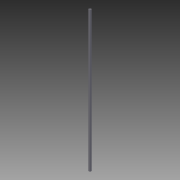
# Autodesk Inventor part: Robot-Mast
Saved by Autodesk Inventor 2012 (Build 160160000, 160)
## iProperties
Created: 2013-07-14
Part Number: Robot-Mast
Material: Aluminum-6061
Document SubType Name: Modeling
Designer: joe_000
Density: 2.71 g/cm^3
Mass: 507.328 g
Surface Area: 2108.26 cm^2
Volume: 187.206 cm^3
MastWidth: 0.750 in
Author: joe_000
Autodesk Inventor part; units mm, degrees
ref_plane "YZ Plane" through (0, 0, 0) normal (1, 0, 0) x (0, 1, 0)
ref_plane "XZ Plane" through (0, 0, 0) normal (0, 1, 0) x (-1, 0, 0)
ref_plane "XY Plane" through (0, 0, 0) normal (0, 0, 1) x (1, 0, 0)
sketch "Sketch1" plane through (0, 0, 0) normal (0, 1, 0) x (-1, 0, 0)
  line L0 (0, 0) -> (19.05, 0)
  line L1 (19.05, 0) -> (19.05, 19.05)
  line L2 (19.05, 19.05) -> (0, 19.05)
  line L3 (0, 19.05) -> (0, 0)
  line L4 (1.778, 17.272) -> (17.272, 17.272)
  line L5 (17.272, 17.272) -> (17.272, 1.778)
  line L6 (17.272, 1.778) -> (1.778, 1.778)
  line L7 (1.778, 1.778) -> (1.778, 17.272)
  dimension "MastWidth" = 19.05
  dimension "d1" = 19.05
  dimension "d2" = 1.778
  dimension "d3" = 1.778
  dimension "d4" = 1.778
  dimension "d5" = 1.778
  constraints: 16 end point, 4 parallel, 2 horizontal, 2 perpendicular
  measures "MastWidth" distance of L1.end L2.end
  measures "d1" distance of L0.end L1.end
  measures "d2" distance between parallel lines of L2 L4
  measures "d3" distance between parallel lines of L3 L7
  measures "d4" distance between parallel lines of L0 L6
  measures "d5" distance between parallel lines of L1 L5
extrude "Extrusion1" add sketch "Sketch1" along normal blind 1524
sketch "Sketch2" plane through (0, 0, 0) normal (0, -1, 0) x (1, 0, 0)
  line L0 (-17.272, 1.778) -> (-17.272, 17.272) projected
  line L1 (-17.272, 17.272) -> (-1.778, 17.272) projected
  line L2 (-1.778, 17.272) -> (-1.778, 1.778) projected
  line L3 (-1.778, 1.778) -> (-17.272, 1.778) projected
  line L4 (0, 0) -> (-19.05, 0) projected
  line L5 (0, 19.05) -> (0, 0) projected
  line L6 (-19.05, 19.05) -> (0, 19.05) projected
  line L7 (-19.05, 0) -> (-19.05, 19.05) projected
  line L8 (-19.05, 9.525) -> (0, 9.525)
  line L9 (-9.525, 19.05) -> (-9.525, 0)
  constraints: 4 end point, 4 midpoint
sketch "Sketch3" plane through (-19.05, 0, 19.05) normal (0, 0, 1) x (1, 0, 0)
  line L0 (19.05, 1524) -> (0, 1524) projected
  line L1 (0, 0) -> (0, 1524) projected
  line L2 (0, 0) -> (19.05, 0) projected
  line L3 (19.05, 0) -> (19.05, 1524) projected
  line L4 (7.0234, 1484.4913) -> (20.0256, 1484.4913) construction
  line L5 (20.0256, 1484.4913) -> (20.0256, 1481.3149) construction
  line L6 (20.0256, 1481.3149) -> (7.0234, 1481.3149) construction
  line L7 (7.0234, 1481.3149) -> (7.0234, 1484.4913) construction
  constraints: 2 other
equation "\"d1\" = MastWidth"
equation "\"d3\" = d2"
equation "\"d4\" = d2"
equation "\"d5\" = d2"
body "Solid1"
